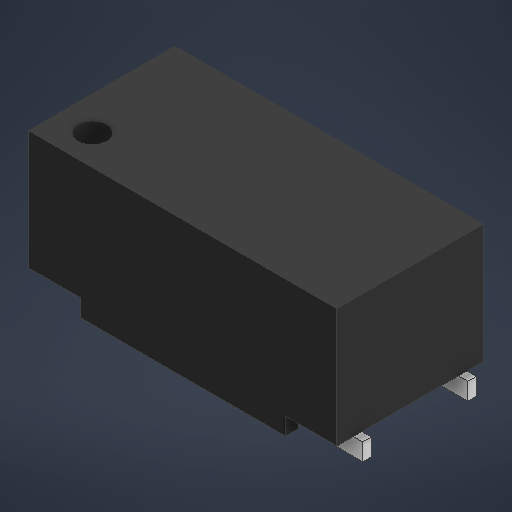
# Autodesk Inventor part: ZS1052_S_HT
Saved by Autodesk Inventor 2026 (Build 300175050, 175E)
## iProperties
Created: 2025-07-31
Part Number: ZS1052_S_HT
Material: Generic
Document SubType Name: Modeling
Designer: user
Density: 1 g/cm^3
Appearance: Default
Author: user
Autodesk Inventor part; units mm, degrees
ref_plane "YZ Plane" through (0, 0, 0) normal (1, 0, 0) x (0, 1, 0)
ref_plane "XZ Plane" through (0, 0, 0) normal (0, 1, 0) x (-1, 0, 0)
ref_plane "XY Plane" through (0, 0, 0) normal (0, 0, 1) x (1, 0, 0)
sketch "Sketch1" plane through (0, 0, 0) normal (0, 1, 0) x (-1, 0, 0)
  line L0 (8.95, -4.25) -> (-8.95, -4.25)
  line L1 (-8.95, -4.25) -> (-8.95, 4.25)
  line L2 (-8.95, 4.25) -> (8.95, 4.25)
  line L3 (8.95, 4.25) -> (8.95, -4.25)
  point P0 (0, 0)
  point P1 (0, -4.25)
  point P2 (-8.95, 0)
  dimension "d0" = 17.9
  dimension "d1" = 8.5
  constraints: 8 end point, 2 midpoint, 2 parallel, 1 horizontal, 1 horizontal alignment, 1 perpendicular, 1 vertical alignment
  measures "d0" distance of L0.start L0.end
  measures "d1" distance of L0.end L1.end
extrude "Extrusion1" add sketch "Sketch1" along normal blind 7.9
sketch "Sketch2" plane through (0, 0, 0) normal (0, -1, 0) x (1, 0, 0)
  line L0 (-8.95, 4.25) -> (8.95, 4.25) projected
  line L1 (-8.95, 4.25) -> (-5.95, 4.25)
  line L2 (-5.95, 4.25) -> (-5.95, -4.25)
  line L3 (-5.95, -4.25) -> (-8.95, -4.25)
  line L4 (-8.95, -4.25) -> (-8.95, 4.25)
  line L5 (8.95, 4.25) -> (5.95, 4.25)
  line L6 (5.95, 4.25) -> (5.95, -4.25)
  line L7 (5.95, -4.25) -> (8.95, -4.25)
  line L8 (8.95, -4.25) -> (8.95, 4.25)
  line L9 (8.95, -4.25) -> (-8.95, -4.25) projected
  line L10 (-5.95, 4.25) -> (5.95, 4.25)
  line L11 (5.95, 4.25) -> (5.95, 3.5)
  line L12 (5.95, 3.5) -> (-5.95, 3.5)
  line L13 (-5.95, 3.5) -> (-5.95, 4.25)
  line L14 (-5.95, -4.25) -> (5.95, -4.25)
  line L15 (5.95, -4.25) -> (5.95, -3.5)
  line L16 (5.95, -3.5) -> (-5.95, -3.5)
  line L17 (-5.95, -3.5) -> (-5.95, -4.25)
  point P0 (0, 0)
  point P1 (-5.95, 3.5)
  dimension "d4" = 3
  dimension "d5" = 3
  dimension "d6" = 0.75
  constraints: 32 end point, 8 parallel, 4 collinear, 4 horizontal, 4 perpendicular, 1 point on line
  measures "d4" distance between parallel lines of L2 L4
  measures "d5" distance between parallel lines of L8 L6
  measures "d6" distance of L10.end L11.end
extrude "Extrusion2" cut sketch "Sketch2" against normal blind 1 contours L0 L2 L3 L4 | L0 L8 L7 L6 | L12 L6 L16 L2
sketch "Sketch3" plane through (0, 0, 0) normal (0, 1, 0) x (-1, 0, 0)
  line L0 (9.5, 2.75) -> (7.7, 2.75)
  line L1 (7.7, 2.75) -> (7.7, 2.25)
  line L2 (7.7, 2.25) -> (9.5, 2.25)
  line L3 (9.5, 2.25) -> (9.5, 2.75)
  line L4 (9.5, -2.25) -> (7.7, -2.25)
  line L5 (7.7, -2.25) -> (7.7, -2.75)
  line L6 (7.7, -2.75) -> (9.5, -2.75)
  line L7 (9.5, -2.75) -> (9.5, -2.25)
  line L8 (9.5, 2.5) -> (9.5, -2.5) construction
  line L9 (-7.7, 3.3) -> (-9.5, 3.3)
  line L10 (-9.5, 3.3) -> (-9.5, 2.8)
  line L11 (-9.5, 2.8) -> (-7.7, 2.8)
  line L12 (-7.7, 2.8) -> (-7.7, 3.3)
  line L13 (-7.7, -2.8) -> (-9.5, -2.8)
  line L14 (-9.5, -2.8) -> (-9.5, -3.3)
  line L15 (-9.5, -3.3) -> (-7.7, -3.3)
  line L16 (-7.7, -3.3) -> (-7.7, -2.8)
  line L17 (-9.5, 3.05) -> (-9.5, -3.05) construction
  line L18 (9.5, 0) -> (-9.5, 0) construction
  point P0 (0, 0)
  point P1 (8.6, -2.25)
  point P2 (8.6, 2.25)
  point P3 (-8.6, -2.8)
  point P4 (-8.6, 2.8)
  point P5 (0, 0)
  dimension "d9" = 0.5
  dimension "d10" = 1.8
  dimension "d11" = 0.5
  dimension "d12" = 1.8
  dimension "d13" = 5
  dimension "d14" = 0.5
  dimension "d15" = 1.8
  dimension "d16" = 0.5
  dimension "d17" = 1.8
  dimension "d19" = 6.1
  dimension "d20" = 19
  constraints: 38 end point, 11 midpoint, 8 parallel, 5 horizontal, 4 perpendicular, 2 vertical alignment, 1 coincident
  measures "d9" distance of L0.end L1.end
  measures "d10" distance of L1.end L2.end
  measures "d11" distance of L4.end L5.end
  measures "d12" distance of L5.end L6.end
  measures "d13" distance of L8.start L8.end
  measures "d14" distance of L9.end L10.end
  measures "d15" distance of L10.end L11.end
  measures "d16" distance of L13.end L14.end
  measures "d17" distance of L14.end L15.end
  measures "d19" distance of L17.start L17.end
  measures "d20" distance of L18.start L18.end
extrude "Extrusion3" add sketch "Sketch3" along normal blind 1
sketch "Sketch4" plane through (0, 7.9, 0) normal (0, 1, 0) x (1, 0, 0)
  circle A0 centre (-7, -2.5) radius 0.8343
  line L0 (-7, -1.6657) -> (-7, -3.3343)
  point P0 (0, 0)
  dimension "d23" = 7
  dimension "d24" = 2.5
  constraints: 2 end point, 2 point on circle, 1 centre point, 1 vertical
  measures "d23" horizontal distance of point (0, 0) A0.centre
  measures "d24" vertical distance of point (0, 0) A0.centre
revolve "Revolution1" cut sketch "Sketch4" angle 360 about axis through (-7, 7.9, 1.6657) along (0, 0, 1) picked at (-6.7647, -2.2895) contours A0 L0
body "Solid1"
